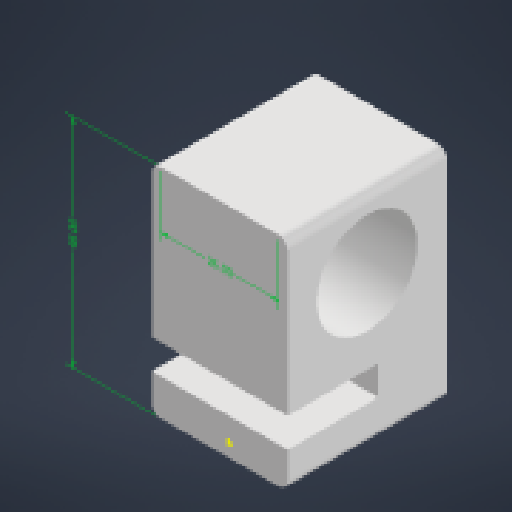
# Autodesk Inventor part: Beltclamp
Saved by Autodesk Inventor 2024.2 (Build 282272000, 272)
## iProperties
Created: 2024-03-09
Part Number: Beltclamp
Material: Generic
Document SubType Name: Modeling
Designer: LightStore
Density: 1 g/cm^3
Appearance: Default
Author: LightStore
Autodesk Inventor part; units mm, degrees
ref_plane "YZ Plane" through (0, 0, 0) normal (1, 0, 0) x (0, 1, 0)
ref_plane "XZ Plane" through (0, 0, 0) normal (0, 1, 0) x (-1, 0, 0)
sketch "Sketch1" plane through (0, 0, 0) normal (0, 0, 1) x (1, 0, 0)
  line L0 (-17.3656, -3.1866) -> (12.6344, -3.1866)
  line L1 (12.6344, -3.1866) -> (12.6344, 9.8134)
  line L2 (12.6344, 9.8134) -> (-17.3656, 9.8134)
  line L3 (-17.3656, 9.8134) -> (-17.3656, -3.1866)
  point P0 (0, 0)
  dimension "d0" = 30
  dimension "d1" = 13
  constraints: 8 end point, 2 parallel, 1 horizontal, 1 perpendicular
  measures "d0" distance of L2.end L1.end
  measures "d1" distance of L1.end L0.end
extrude "Extrusion1" add sketch "Sketch1" along normal blind 35
sketch "Sketch2" plane through (0, 0, 35) normal (0, 0, 1) x (1, 0, 0)
  point P0 (0, 0)
sketch "Sketch3" plane through (0, 0, 35) normal (0, 0, 1) x (1, 0, 0)
  line L0 (-24.8388, 28.6624) -> (-24.5328, 28.6624)
  line L1 (12.6344, -3.1866) -> (12.6344, 9.8134) projected
  line L2 (-17.3656, 9.8134) -> (-17.3656, -3.1866) projected
  line L3 (-17.3656, 11.3273) -> (-17.3656, 4.8273)
  line L4 (15.1579, 11.3273) -> (15.1579, 4.8273)
  line L5 (-17.3656, 4.8273) -> (15.1579, 4.8273)
  line L6 (-17.3656, 11.3273) -> (15.1579, 11.3273)
  line L7 (-43.7964, 23.1681) -> (-44.8479, 23.9265)
  line L8 (-44.8479, 23.9265) -> (-43.7964, 23.1681)
  line L9 (-42.6813, 23.9265) -> (-43.7964, 23.1681)
  line L10 (-44.8479, 23.9265) -> (-45.923, 23.1739)
  line L11 (-41.5979, 23.1681) -> (-42.6813, 23.9265)
  line L12 (-40.5146, 23.9265) -> (-41.5979, 23.1681)
  line L13 (-38.3479, 23.9265) -> (-37.2646, 23.1681)
  line L14 (-37.2646, 23.1681) -> (-38.3479, 23.9265)
  line L15 (-40.5146, 23.9265) -> (-39.4313, 23.1681)
  line L16 (-38.3479, 23.9265) -> (-39.4313, 23.1681)
  line L17 (-39.4313, 23.1681) -> (-40.5146, 23.9265)
  line L18 (-30.7646, 23.1681) -> (-29.6813, 23.9265)
  line L19 (-29.6813, 23.9265) -> (-30.7646, 23.1681)
  line L20 (-31.8479, 23.9265) -> (-30.7646, 23.1681)
  line L21 (-32.9313, 23.1681) -> (-31.8479, 23.9265)
  line L22 (-36.1813, 23.9265) -> (-35.0979, 23.1681)
  line L23 (-34.0146, 23.9265) -> (-35.0979, 23.1681)
  line L24 (-35.0979, 23.1681) -> (-34.0146, 23.9265)
  line L25 (-34.0146, 23.9265) -> (-32.9313, 23.1681)
  line L26 (-36.1813, 23.9265) -> (-37.2646, 23.1681)
  line L27 (-29.6813, 23.9265) -> (-28.5979, 23.1681)
  line L28 (-14.5146, 23.9265) -> (-13.3995, 23.1739)
  line L29 (-15.5979, 23.1681) -> (-14.5146, 23.9265)
  line L30 (-16.6813, 23.9265) -> (-15.5979, 23.1681)
  line L31 (-16.6813, 23.9265) -> (-17.7646, 23.1681)
  line L32 (-17.7646, 23.1681) -> (-16.6813, 23.9265)
  line L33 (-18.8479, 23.9265) -> (-17.7646, 23.1681)
  line L34 (-18.8479, 23.9265) -> (-19.9313, 23.1681)
  line L35 (-19.9313, 23.1681) -> (-18.8479, 23.9265)
  line L36 (-21.0146, 23.9265) -> (-19.9313, 23.1681)
  line L37 (-21.0146, 23.9265) -> (-22.0979, 23.1681)
  line L38 (-23.1813, 23.9265) -> (-22.0979, 23.1681)
  line L39 (-22.0979, 23.1681) -> (-23.1813, 23.9265)
  line L40 (-23.1813, 23.9265) -> (-24.2646, 23.1681)
  line L41 (-24.2646, 23.1681) -> (-25.3479, 23.9265)
  line L42 (-26.4313, 23.1681) -> (-27.5146, 23.9265)
  line L43 (-27.5146, 23.9265) -> (-26.4313, 23.1681)
  line L44 (-25.3479, 23.9265) -> (-26.4313, 23.1681)
  line L45 (-27.5146, 23.9265) -> (-28.5979, 23.1681)
  line L46 (-45.923, 23.1739) -> (-45.923, 16.6739)
  line L47 (-13.3995, 23.1739) -> (-13.3995, 16.6739)
  line L48 (-45.923, 16.6739) -> (-13.3995, 16.6739)
  line L49 (-45.923, 23.1739) -> (-13.3995, 23.1739)
  point P0 (-17.3656, 7.8134)
  point P1 (10.6344, 9.8134)
  point P2 (-15.3656, 9.8134)
  point P3 (-17.3656, 2.7291)
  point P4 (15.1344, 5.7756)
  point P5 (-17.3656, 5.5444)
  point P6 (-17.3656, 2.7304)
  point P7 (12.6344, 4.8273)
  point P8 (-17.3656, 9.8134)
  point P9 (-45.923, 19.66)
  point P10 (-17.923, 21.66)
  point P11 (-43.923, 21.66)
  point P12 (-45.923, 21.66)
  point P13 (-15.923, 21.66)
  point P14 (-37.2646, 23.1828)
  point P15 (-19.9313, 23.1828)
  point P16 (-45.923, 17.391)
  dimension "d79" = 6.5
  constraints: 96 end point, 3 horizontal, 2 parallel, 1 perpendicular
  measures "d79" distance of L10.end L48.start
fillet "Fillet2" radius 2 2 edges at (-17.3656, -3.1866, 17.5) (12.6344, -3.1866, 17.5)
sketch "Sketch5" plane through (0, 0, 35) normal (0, 0, 1) x (1, 0, 0)
  line L0 (-17.3656, 0.1134) -> (-17.3656, 5.1134) projected
  line L1 (-17.3656, 21.8134) -> (-17.3656, 25.9634) construction
  line L2 (12.6344, 9.8134) -> (-17.3656, 9.8134) construction
  line L3 (-17.3656, 44.8134) -> (12.6344, 44.8134)
  line L4 (12.6344, 21.8134) -> (12.6344, 44.8134)
  line L5 (-17.3656, 9.8134) -> (12.6344, 9.8134) construction
  line L6 (-17.3656, 21.8134) -> (-17.3656, 44.8134)
  line L7 (12.6344, 9.8134) -> (-17.3656, 9.8134)
  line L8 (-17.3656, 21.8134) -> (-17.3656, 9.8134)
  line L9 (12.6344, 21.8134) -> (12.6344, 9.8134)
  line L10 (12.6344, 9.8134) -> (2.6344, 9.8134)
  point P0 (0, 0)
  point P1 (-17.3656, 2.6134)
  dimension "d15" = 23.35
  dimension "d17" = 35
  dimension "d20" = 30
  dimension "d21" = 10
  constraints: 19 end point, 4 collinear, 4 point on line, 1 horizontal, 1 midpoint, 1 perpendicular, 1 vertical
  measures "d15" distance of point (-17.366, 2.613) L1.end
  measures "d17" distance of L2.end L3.start
  measures "d20" distance of L2.end L5.end
  measures "d21" distance of L2.start L10.end
extrude "Extrusion4" add sketch "Sketch5" against normal blind 35
ref_plane "Work Plane4" through (-17.3656, 0.1134, 28.8) normal (-1, 0, 0) x (0, 0, 1)
sketch "Sketch6" plane through (-17.3656, 0.1134, 28.8) normal (-1, 0, 0) x (0, 0, 1)
  line L0 (6.2, 44.7) -> (6.2, 5) projected
  line L1 (6.2, 29.7) -> (-11.3, 29.7) construction
  line L2 (6.2, 29.7) -> (23.7, 29.7) construction
  circle A0 centre (-11.3, 29.7) radius 11.1
  line L3 (6.2, 44.7) -> (-28.8, 44.7) projected
  point P0 (-28.8, -0.1134)
  point P1 (6.2, 27.7)
  dimension "d24" = 17.5
  dimension "d25" = 180
  dimension "d26" = 22.2
  dimension "d58" = 15
  constraints: 4 end point, 1 centre point, 1 coincident, 1 collinear, 1 horizontal, 1 perpendicular, 1 point on line
  measures "d24" distance of L1.start L1.end
  measures "d25" angle of L1 L2
  measures "d26" diameter of A0
  measures "d58" distance from line of L1.end L3
fillet "Fillet3" radius 2 2 edges at (-17.3656, 44.8134, 17.5) (12.6344, 44.8134, 17.5)
extrude "Extrusion7" cut sketch "Sketch6" against normal blind 35
sketch "Sketch8" plane through (0, 0, 0) normal (0, 0, -1) x (-1, 0, 0)
  circle A0 centre (-4.6344, 11.0711) radius 1.5 projected
  circle A1 centre (-4.6344, 11.0711) radius 1.5
  circle A2 centre (-4.6344, 16.0711) radius 1.5 projected
  circle A3 centre (-4.6344, 16.0711) radius 1.5
  circle A4 centre (9.3656, 16.0711) radius 1.5 projected
  circle A5 centre (9.3656, 16.0711) radius 1.5
  circle A6 centre (9.3656, 11.0711) radius 1.5 projected
  circle A7 centre (9.3656, 11.0711) radius 1.5
  point P0 (0, 0)
  constraints: 4 centre point, 4 coincident
extrude "Extrusion8" cut sketch "Sketch8" against normal blind 10
sketch "Sketch9" plane through (0, 0, 35) normal (0, 0, 1) x (1, 0, 0)
  point P0 (0, 0)
extrude "Extrusion14" cut sketch "Sketch3" against normal blind 30 contours L3 L6 L4 L5 L2
thread "Thread1" size "M3x0.5" class "6H" standard "ANSI Metric M Profile" full length
thread "Thread2" size "M3x0.5" class "6H" standard "ANSI Metric M Profile" full length
thread "Thread3" size "M3x0.5" class "6H" standard "ANSI Metric M Profile" full length
thread "Thread4" size "M3x0.5" class "6H" standard "ANSI Metric M Profile" full length
body "Solid1"
